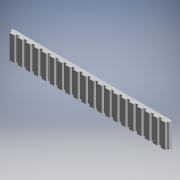
# Autodesk Inventor part: HTBO-S5M150-616
Saved by Autodesk Inventor 2017.3 (Build 213256000, 256)
## iProperties
Part Number: HTBO-S5M150-616
Material: Generic
Catalog Web Link: www.cadenas.de
Description: HTBO-S3M, HTBO-S5M, HTBO-S8M, HTBOG-S5M, HTBOG-S8M-Open End Belts - S Type
Vendor: MISUMI
Document SubType Name: Modeling
Designer: partserver
Manufacturer: MISUMI
Mass: 4.10999 g
Surface Area: 42.6466 cm^2
Volume: 4.10999 cm^3
Density: 1 g/cm^3
Appearance: PSOLRGB-234-234-234
Category: PARTsolutions
Company: MISUMI
Title: HTBO-S5M150-616
Author: Cadenas PARTsolutions
Comments: Open End Belts - S Type
PSOL_IDENT_0: {$CADENAS_DATA\23d-libs\misumi\metric\48_timing_belts\htbog_s5m.prj},228 {VTYP=3D},{NB=HTBO-S5M150-6
PSOL_IDENT_1: 16},{LINA=HTBO-S5M150-616},{NN=HTBO-S3M, HTBO-S5M, HTBO-S8M, HTBOG-S5M, HTBOG-S8M},{DATE=30.06.2021
PSOL_IDENT_2: 13:24:08},{GEOMDATE=28.08.2009 09:14:00},{VERSION=},{LINEID=40},{WBVAR=MATMB,BNW,NT},{WBNUMERIC=NT}
PSOL_IDENT_3: {NB=HTBO-S5M150-616},{LINA=HTBO-S5M150-616},{KT=DUMMY},{PN=HTBO-S5M150-616},{MATMB=},{MATMBALG=  'G'
PSOL_IDENT_4: ,'Chloroprene Rubber','','Polyurethane'                       },{MATCW=Steel Cord},{COLOR=White},{OT=
PSOL_IDENT_5: -20~80},{TB=S5M},{BNW=150},{NT=616},{BW=15},{AT=323},{MAX=20},{AMJ=TBCK-S5M150},{PITCH=5},{RAA=3.25}
PSOL_IDENT_6: ,{LRR=3.25},{H=3.20},{HH=1.77},{II=2.00},{PLD=0.480},{UM=34.6},{BNWALG= '100','100','150','150','250'
PSOL_IDENT_7: ,'250'},{NTALG=[50:4000]},{NOTE=3D Model is Only a Segment of the Actual Belt},{COL=0.92,0.92,0.92,0
PSOL_IDENT_8: .00}
NB: HTBO-S5M150-616
NN: HTBO-S3M, HTBO-S5M, HTBO-S8M, HTBOG-S5M, HTBOG-S8M
NT: 616
NBSYN: $PN.
LINA: HTBO-S5M150-616
CATALOG: Misumi
PN: HTBO-S5M150-616
MATMB: Polyurethane
MATCW: Steel Cord
COLOR: White
OT: -20~80
TB: S5M
BNW: 150
BW: 15
AT: 323
AMJ: TBCK-S5M150
PITCH: 5
RAA: 3.25
LRR: 3.25
H: 3.2
HH: 1.77
II: 2
PLD: 0.48
UM: 34.6
NOTE: 3D Model is Only a Segment of the Actual Belt
SUPPLIER: MISUMI
ARTICLENO: HTBO-S5M150-616
BOMINFO: HTBO-S5M150-616
CREATOR: CADENAS GmbH
Autodesk Inventor part; units mm, degrees
ref_plane "YZ Plane" through (0, 0, 0) normal (1, 0, 0) x (0, 1, 0)
ref_plane "XZ Plane" through (0, 0, 0) normal (0, 1, 0) x (-1, 0, 0)
ref_plane "XY Plane" through (0, 0, 0) normal (0, 0, 1) x (1, 0, 0)
sketch "Sketch_1" plane through (0, 0, 0) normal (0, 0, 1) x (1, 0, 0)
  line L0 (-5, 1) -> (-5, -1)
  line L1 (-5, -1) -> (-4.125, -1)
  arc A0 (-4.125, -1) -> (-3.8953, -2.2) centre (-0.875, -1) ccw
  line L2 (-3.8953, -2.2) -> (-1.1047, -2.2)
  arc A1 (-1.1047, -2.2) -> (-0.875, -1) centre (-4.125, -1) ccw
  line L3 (-0.875, -1) -> (-0.1, -1)
  line L4 (-0.1, -1) -> (-0.1, -0.9)
  line L5 (-0.1, -0.9) -> (0.1, -0.9)
  line L6 (0.1, -0.9) -> (0.1, -1)
  line L7 (0.1, -1) -> (0.875, -1)
  arc A2 (0.875, -1) -> (1.1047, -2.2) centre (4.125, -1) ccw
  line L8 (1.1047, -2.2) -> (3.8953, -2.2)
  arc A3 (3.8953, -2.2) -> (4.125, -1) centre (0.875, -1) ccw
  line L9 (4.125, -1) -> (4.9, -1)
  line L10 (4.9, -1) -> (4.9, -0.9)
  line L11 (4.9, -0.9) -> (5.1, -0.9)
  line L12 (5.1, -0.9) -> (5.1, -1)
  line L13 (5.1, -1) -> (5.875, -1)
  arc A4 (5.875, -1) -> (6.1047, -2.2) centre (9.125, -1) ccw
  line L14 (6.1047, -2.2) -> (8.8953, -2.2)
  arc A5 (8.8953, -2.2) -> (9.125, -1) centre (5.875, -1) ccw
  line L15 (9.125, -1) -> (9.9, -1)
  line L16 (9.9, -1) -> (9.9, -0.9)
  line L17 (9.9, -0.9) -> (10.1, -0.9)
  line L18 (10.1, -0.9) -> (10.1, -1)
  line L19 (10.1, -1) -> (10.875, -1)
  arc A6 (10.875, -1) -> (11.1047, -2.2) centre (14.125, -1) ccw
  line L20 (11.1047, -2.2) -> (13.8953, -2.2)
  arc A7 (13.8953, -2.2) -> (14.125, -1) centre (10.875, -1) ccw
  line L21 (14.125, -1) -> (14.9, -1)
  line L22 (14.9, -1) -> (14.9, -0.9)
  line L23 (14.9, -0.9) -> (15.1, -0.9)
  line L24 (15.1, -0.9) -> (15.1, -1)
  line L25 (15.1, -1) -> (15.875, -1)
  arc A8 (15.875, -1) -> (16.1047, -2.2) centre (19.125, -1) ccw
  line L26 (16.1047, -2.2) -> (18.8953, -2.2)
  arc A9 (18.8953, -2.2) -> (19.125, -1) centre (15.875, -1) ccw
  line L27 (19.125, -1) -> (19.9, -1)
  line L28 (19.9, -1) -> (19.9, -0.9)
  line L29 (19.9, -0.9) -> (20.1, -0.9)
  line L30 (20.1, -0.9) -> (20.1, -1)
  line L31 (20.1, -1) -> (20.875, -1)
  arc A10 (20.875, -1) -> (21.1047, -2.2) centre (24.125, -1) ccw
  line L32 (21.1047, -2.2) -> (23.8953, -2.2)
  arc A11 (23.8953, -2.2) -> (24.125, -1) centre (20.875, -1) ccw
  line L33 (24.125, -1) -> (24.9, -1)
  line L34 (24.9, -1) -> (24.9, -0.9)
  line L35 (24.9, -0.9) -> (25.1, -0.9)
  line L36 (25.1, -0.9) -> (25.1, -1)
  line L37 (25.1, -1) -> (25.875, -1)
  arc A12 (25.875, -1) -> (26.1047, -2.2) centre (29.125, -1) ccw
  line L38 (26.1047, -2.2) -> (28.8953, -2.2)
  arc A13 (28.8953, -2.2) -> (29.125, -1) centre (25.875, -1) ccw
  line L39 (29.125, -1) -> (29.9, -1)
  line L40 (29.9, -1) -> (29.9, -0.9)
  line L41 (29.9, -0.9) -> (30.1, -0.9)
  line L42 (30.1, -0.9) -> (30.1, -1)
  line L43 (30.1, -1) -> (30.875, -1)
  arc A14 (30.875, -1) -> (31.1047, -2.2) centre (34.125, -1) ccw
  line L44 (31.1047, -2.2) -> (33.8953, -2.2)
  arc A15 (33.8953, -2.2) -> (34.125, -1) centre (30.875, -1) ccw
  line L45 (34.125, -1) -> (34.9, -1)
  line L46 (34.9, -1) -> (34.9, -0.9)
  line L47 (34.9, -0.9) -> (35.1, -0.9)
  line L48 (35.1, -0.9) -> (35.1, -1)
  line L49 (35.1, -1) -> (35.875, -1)
  arc A16 (35.875, -1) -> (36.1047, -2.2) centre (39.125, -1) ccw
  line L50 (36.1047, -2.2) -> (38.8953, -2.2)
  arc A17 (38.8953, -2.2) -> (39.125, -1) centre (35.875, -1) ccw
  line L51 (39.125, -1) -> (39.9, -1)
  line L52 (39.9, -1) -> (39.9, -0.9)
  line L53 (39.9, -0.9) -> (40.1, -0.9)
  line L54 (40.1, -0.9) -> (40.1, -1)
  line L55 (40.1, -1) -> (40.875, -1)
  arc A18 (40.875, -1) -> (41.1047, -2.2) centre (44.125, -1) ccw
  line L56 (41.1047, -2.2) -> (43.8953, -2.2)
  arc A19 (43.8953, -2.2) -> (44.125, -1) centre (40.875, -1) ccw
  line L57 (44.125, -1) -> (44.9, -1)
  line L58 (44.9, -1) -> (44.9, -0.9)
  line L59 (44.9, -0.9) -> (45.1, -0.9)
  line L60 (45.1, -0.9) -> (45.1, -1)
  line L61 (45.1, -1) -> (45.875, -1)
  arc A20 (45.875, -1) -> (46.1047, -2.2) centre (49.125, -1) ccw
  line L62 (46.1047, -2.2) -> (48.8953, -2.2)
  arc A21 (48.8953, -2.2) -> (49.125, -1) centre (45.875, -1) ccw
  line L63 (49.125, -1) -> (49.9, -1)
  line L64 (49.9, -1) -> (49.9, -0.9)
  line L65 (49.9, -0.9) -> (50.1, -0.9)
  line L66 (50.1, -0.9) -> (50.1, -1)
  line L67 (50.1, -1) -> (50.875, -1)
  arc A22 (50.875, -1) -> (51.1047, -2.2) centre (54.125, -1) ccw
  line L68 (51.1047, -2.2) -> (53.8953, -2.2)
  arc A23 (53.8953, -2.2) -> (54.125, -1) centre (50.875, -1) ccw
  line L69 (54.125, -1) -> (54.9, -1)
  line L70 (54.9, -1) -> (54.9, -0.9)
  line L71 (54.9, -0.9) -> (55.1, -0.9)
  line L72 (55.1, -0.9) -> (55.1, -1)
  line L73 (55.1, -1) -> (55.875, -1)
  arc A24 (55.875, -1) -> (56.1047, -2.2) centre (59.125, -1) ccw
  line L74 (56.1047, -2.2) -> (58.8953, -2.2)
  arc A25 (58.8953, -2.2) -> (59.125, -1) centre (55.875, -1) ccw
  line L75 (59.125, -1) -> (59.9, -1)
  line L76 (59.9, -1) -> (59.9, -0.9)
  line L77 (59.9, -0.9) -> (60.1, -0.9)
  line L78 (60.1, -0.9) -> (60.1, -1)
  line L79 (60.1, -1) -> (60.875, -1)
  arc A26 (60.875, -1) -> (61.1047, -2.2) centre (64.125, -1) ccw
  line L80 (61.1047, -2.2) -> (63.8953, -2.2)
  arc A27 (63.8953, -2.2) -> (64.125, -1) centre (60.875, -1) ccw
  line L81 (64.125, -1) -> (64.9, -1)
  line L82 (64.9, -1) -> (64.9, -0.9)
  line L83 (64.9, -0.9) -> (65.1, -0.9)
  line L84 (65.1, -0.9) -> (65.1, -1)
  line L85 (65.1, -1) -> (65.875, -1)
  arc A28 (65.875, -1) -> (66.1047, -2.2) centre (69.125, -1) ccw
  line L86 (66.1047, -2.2) -> (68.8953, -2.2)
  arc A29 (68.8953, -2.2) -> (69.125, -1) centre (65.875, -1) ccw
  line L87 (69.125, -1) -> (69.9, -1)
  line L88 (69.9, -1) -> (69.9, -0.9)
  line L89 (69.9, -0.9) -> (70.1, -0.9)
  line L90 (70.1, -0.9) -> (70.1, -1)
  line L91 (70.1, -1) -> (70.875, -1)
  arc A30 (70.875, -1) -> (71.1047, -2.2) centre (74.125, -1) ccw
  line L92 (71.1047, -2.2) -> (73.8953, -2.2)
  arc A31 (73.8953, -2.2) -> (74.125, -1) centre (70.875, -1) ccw
  line L93 (74.125, -1) -> (74.9, -1)
  line L94 (74.9, -1) -> (74.9, -0.9)
  line L95 (74.9, -0.9) -> (75.1, -0.9)
  line L96 (75.1, -0.9) -> (75.1, -1)
  line L97 (75.1, -1) -> (75.875, -1)
  arc A32 (75.875, -1) -> (76.1047, -2.2) centre (79.125, -1) ccw
  line L98 (76.1047, -2.2) -> (78.8953, -2.2)
  arc A33 (78.8953, -2.2) -> (79.125, -1) centre (75.875, -1) ccw
  line L99 (79.125, -1) -> (79.9, -1)
  line L100 (79.9, -1) -> (79.9, -0.9)
  line L101 (79.9, -0.9) -> (80.1, -0.9)
  line L102 (80.1, -0.9) -> (80.1, -1)
  line L103 (80.1, -1) -> (80.875, -1)
  arc A34 (80.875, -1) -> (81.1047, -2.2) centre (84.125, -1) ccw
  line L104 (81.1047, -2.2) -> (83.8953, -2.2)
  arc A35 (83.8953, -2.2) -> (84.125, -1) centre (80.875, -1) ccw
  line L105 (84.125, -1) -> (84.9, -1)
  line L106 (84.9, -1) -> (84.9, -0.9)
  line L107 (84.9, -0.9) -> (85.1, -0.9)
  line L108 (85.1, -0.9) -> (85.1, -1)
  line L109 (85.1, -1) -> (85.875, -1)
  arc A36 (85.875, -1) -> (86.1047, -2.2) centre (89.125, -1) ccw
  line L110 (86.1047, -2.2) -> (88.8953, -2.2)
  arc A37 (88.8953, -2.2) -> (89.125, -1) centre (85.875, -1) ccw
  line L111 (89.125, -1) -> (89.9, -1)
  line L112 (89.9, -1) -> (89.9, -0.9)
  line L113 (89.9, -0.9) -> (90.1, -0.9)
  line L114 (90.1, -0.9) -> (90.1, -1)
  line L115 (90.1, -1) -> (90.875, -1)
  arc A38 (90.875, -1) -> (91.1047, -2.2) centre (94.125, -1) ccw
  line L116 (91.1047, -2.2) -> (93.8953, -2.2)
  arc A39 (93.8953, -2.2) -> (94.125, -1) centre (90.875, -1) ccw
  line L117 (94.125, -1) -> (95, -1)
  line L118 (95, -1) -> (95, 1)
  line L119 (95, 1) -> (-5, 1)
  constraints: 240 end point, 80 point on circle, 40 centre point
extrude "Extrusion1" add sketch "Sketch_1" along normal mid plane 15
body "Solid1"
